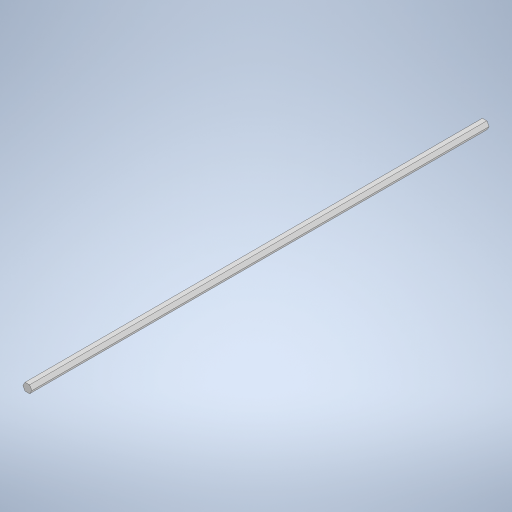
# Autodesk Inventor part: 4-bar intake shaft (29.5)
Saved by Autodesk Inventor 2023 (Build 270158030, 158C)
## iProperties
Created: 2022-07-21
Part Number: 4-bar intake shaft (29.5)
Material: Generic
Document SubType Name: Modeling
Designer: rm0990889
Density: 1 g/cm^3
Appearance: Default
Author: rm0990889
Autodesk Inventor part; units mm, degrees
ref_plane "YZ Plane" through (0, 0, 0) normal (1, 0, 0) x (0, 1, 0)
ref_plane "XZ Plane" through (0, 0, 0) normal (0, 1, 0) x (-1, 0, 0)
ref_plane "XY Plane" through (0, 0, 0) normal (0, 0, 1) x (1, 0, 0)
sketch "Sketch1" plane through (0, 0, 0) normal (0, 0, 1) x (1, 0, 0)
  circle A0 centre (0, 0) radius 6.35
  line L0 (7.3323, -0.0033) -> (3.6633, -6.3517)
  line L1 (3.6633, -6.3517) -> (-3.6691, -6.3483)
  line L2 (-3.6691, -6.3483) -> (-7.3323, 0.0033)
  line L3 (-7.3323, 0.0033) -> (-3.6633, 6.3517)
  line L4 (-3.6633, 6.3517) -> (3.6691, 6.3483)
  line L5 (3.6691, 6.3483) -> (7.3323, -0.0033)
  point P0 (5.5007, 3.1725)
  dimension "d0" = 12.7
  constraints: 12 end point, 2 coincident, 1 midpoint, 16 other
extrude "Extrusion1" add sketch "Sketch1" along normal blind 749.3
body "Solid1"
